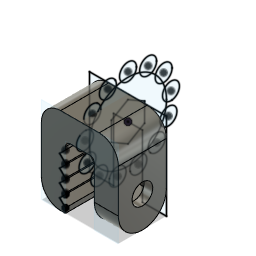
Filament Clip v3 (Autodesk Fusion 360 design; units mm, degrees)
Autodesk Fusion 360 part; units mm, degrees
sketch "Sketch1" plane through (0, 0, 0) normal (0, 0, 1) x (1, 0, 0)
  line L0 (-3, -13) -> (-8, -13)
  line L1 (-8, -13) -> (-8, 5)
  line L2 (-8, 5) -> (8, 5)
  line L3 (8, 5) -> (8, -13)
  line L4 (8, -13) -> (3, -13)
  line L5 (3, -13) -> (3, 0)
  line L6 (3, 0) -> (-3, 0)
  line L7 (-3, 0) -> (-3, -13)
  dimension "d1" = 6
  dimension "d2" = 5
  dimension "d3" = 5
  dimension "d4" = 5
  dimension "d6" = 13
  constraint horizontal L0
  constraint perpendicular L0 L1
  constraint perpendicular L1 L2
  constraint perpendicular L0 L3
  constraint perpendicular L1 L4
  constraint perpendicular L4 L5
  constraint perpendicular L5 L6
  constraint perpendicular L0 L7
  constraint midpoint L6 origin
  constraint collinear L0 L4
  measures "d1" distance of L5.end L6.end
  measures "d2" distance of L0.start L0.end
  measures "d3" distance of L3.end L4.end
  measures "d4" distance of L2 L6
  measures "d6" distance of L4.end L5.end
extrude "Extrude1" add sketch "Sketch1" along normal blind 10 makes body 1
sketch "Sketch2" plane through (3, 0, 0) normal (-1, 0, 0) x (0, 0, 1)
  line L0 (0, 0) -> (0, -13)
  line L1 (0, -13) -> (10, -13)
  line L2 (10, -13) -> (10, 0)
  line L3 (10, 0) -> (0, 0)
  line L4 (8.45, -8.4919) -> (8.45, -4.5081)
  line L5 (8.45, -4.5081) -> (5, -2.5163)
  line L6 (5, -2.5163) -> (1.55, -4.5081)
  line L7 (1.55, -4.5081) -> (1.55, -8.4919)
  line L8 (1.55, -8.4919) -> (5, -10.4837)
  line L9 (5, -10.4837) -> (8.45, -8.4919)
  point P0 (5, -6.5)
  point P1 (5, 0)
  dimension "d9" = 3.45
  dimension "d10" = 6.5
  constraint midpoint L3 P1
  constraint vertical P0 P1
  constraint parallel L0 L7
  measures "d9" distance of P0 L9
  measures "d10" distance of L1 P0
extrude "Extrude2" cut sketch "Sketch2" against normal blind 3.2 contours L4 L5 L6 L7 L8 L9 bodies 1
hole "Hole1" at (3, -6.5, 5) direction (1, 0, 0) diameter 4.3 end through all bodies 1
sketch "Sketch3" plane through (0, 0, 0) normal (1, 0, 0) x (0, 0, -1)
  circle A0 centre (0, 0) radius 8
  line L0 (0, -3.9837) -> (3.45, -1.9919)
  line L1 (3.45, -1.9919) -> (3.45, 1.9919)
  line L2 (3.45, 1.9919) -> (0, 3.9837)
  line L3 (0, 3.9837) -> (-3.45, 1.9919)
  line L4 (-3.45, 1.9919) -> (-3.45, -1.9919)
  line L5 (-3.45, -1.9919) -> (0, -3.9837)
  circle A1 centre (0, 9) radius 1.75
  circle A2 centre (-4.1825, 7.9691) radius 1.75
  circle A3 centre (-7.4069, 5.1126) radius 1.75
  circle A4 centre (-8.9344, 1.0848) radius 1.75
  circle A5 centre (-8.4151, -3.1914) radius 1.75
  circle A6 centre (-5.9681, -6.7366) radius 1.75
  circle A7 centre (-2.1538, -8.7385) radius 1.75
  circle A8 centre (2.1538, -8.7385) radius 1.75
  circle A9 centre (5.9681, -6.7366) radius 1.75
  circle A10 centre (8.4151, -3.1914) radius 1.75
  circle A11 centre (8.9344, 1.0848) radius 1.75
  circle A12 centre (7.4069, 5.1126) radius 1.75
  circle A13 centre (4.1825, 7.9691) radius 1.75
  dimension "d16" = 16
  dimension "d17" = 3.45
  dimension "d18" = 3.5
  dimension "d19" = 9
  dimension "d21" = 360
  constraint coincident A0.centre origin
  constraint vertical A0.centre L2.end
  constraint vertical A0.centre A1.centre
  measures "d16" diameter of A0
  measures "d17" distance of A0.centre L5
  measures "d18" diameter of A1
  measures "d19" distance of A0.centre A1.centre
extrude "Extrude3" add sketch "Sketch3" along normal blind 5 separate body contours A0 A1 A2 A3 A4 A5 A6 A7 A8 A9 A10 A11 A12 A13 | L0 L1 L2 L3 L4 L5 makes body 2
extrude "Extrude4" cut sketch "Sketch3" along normal blind 3 contours L0 L1 L2 L3 L4 L5 bodies 2
hole "Hole2" at (0, 0, 0) direction (1, 0, 0) diameter 4.2 end through all bodies 2
sketch "Sketch4" plane through (0, 0, 10) normal (0, 0, 1) x (1, 0, 0)
  line L0 (-3, 0) -> (3, 0)
  line L1 (3, 0) -> (3, -13)
  line L2 (3, -13) -> (8, -13)
  line L3 (8, -13) -> (8, 5)
  line L4 (8, 5) -> (-8, 5)
  line L5 (-8, 5) -> (-8, -13)
  line L6 (-8, -13) -> (-3, -13)
  line L7 (-3, -13) -> (-3, 0)
  line L8 (-3, -12) -> (-4.2, -10.8)
  line L9 (-4.2, -10.8) -> (-3, -9.6)
  line L10 (-4.2, -8.1333) -> (-3, -6.9333)
  line L11 (-3, -9.3333) -> (-4.2, -8.1333)
  line L12 (-4.2, -5.4667) -> (-3, -4.2667)
  line L13 (-3, -6.6667) -> (-4.2, -5.4667)
  line L14 (-4.2, -2.8) -> (-3, -1.6)
  line L15 (-3, -4) -> (-4.2, -2.8)
  dimension "d29" = 1.2
  dimension "d30" = 1
  dimension "d33" = 0
  dimension "d34" = 8
  constraint coincident L7 L8.start
  constraint coincident L7 L9.end
  constraint equal L8 L9
  constraint perpendicular L8 L9
  measures "d29" distance of L7 L8.end
  measures "d30" distance of L6.end L8.start
extrude "Extrude5" cut sketch "Sketch4" against normal through all contours L7 L14 L15 | L7 L12 L13 | L7 L10 L11 | L7 L8 L9 bodies 1
fillet "Fillet2" radius 5 2 edges at (5.5, -13, 10) (5.5, -13, 0) on bodies 1
fillet "Fillet1" radius 4 3 edges at (-8, 5, 5) (8, 5, 5) (-8, -13, 5) on bodies 1
fillet "Fillet1" radius 1 2 edges at (-3, 0, 5) (3, 0, 5) on bodies 1
fillet "Fillet3" radius 1 26 edges at (0, 4.1185, 5.9666) (0, 2.8368, 7.4801) (0, 0.8739, 7.1971) (0, -0.9643, 7.9417) (0, -2.5709, 6.7789) (0, -4.5445, 6.5839) (0, -5.4267, 4.8076) (0, -7.0836, 3.7178) (0, -7.0393, 1.735) (0, -8, 0) (0, -7.0393, -1.735) (0, -7.0836, -3.7178) (0, -5.4267, -4.8076) (0, -4.5445, -6.5839) (0, -2.5709, -6.7789) (0, -0.9643, -7.9417) (0, 0.8739, -7.1971) (0, 2.8368, -7.4801) (0, 4.1185, -5.9666) (0, 5.9881, -5.305) (0, 6.4196, -3.3692) (0, 7.7675, -1.9145) (0, 7.25, 0) (0, 7.7675, 1.9145) (0, 6.4196, 3.3692) (0, 5.9881, 5.305) on bodies 2
hidden bodies 2
equation "d9 = ( 6.9 / 2 ) * 1 mm"
named bodies: "Tělo", "Matice"
